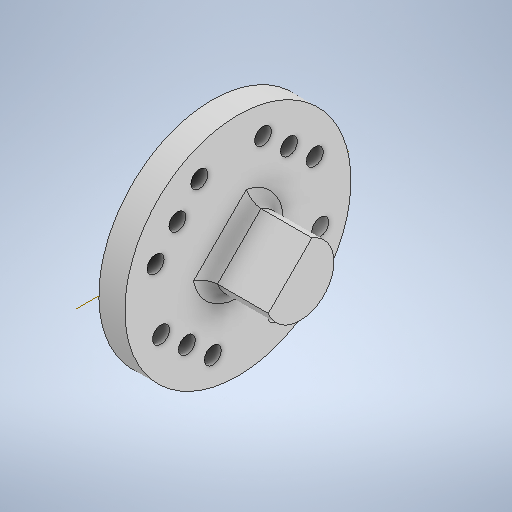
# Autodesk Inventor part: Printed Horn
Saved by Autodesk Inventor 2025.2 (Build 292293000, 293)
## iProperties
Created: 2025-04-05
Part Number: Printed Horn
Material: Generic
Document SubType Name: Modeling
Designer: abdal
Density: 1 g/cm^3
Appearance: Default
Author: abdal
Autodesk Inventor part; units mm, degrees
ref_plane "YZ Plane" through (0, 0, 0) normal (1, 0, 0) x (0, 1, 0)
ref_plane "XZ Plane" through (0, 0, 0) normal (0, 1, 0) x (-1, 0, 0)
ref_plane "XY Plane" through (0, 0, 0) normal (0, 0, 1) x (1, 0, 0)
sketch "Sketch1" plane through (0, 0, 0) normal (1, 0, 0) x (0, 1, 0)
  circle A0 centre (0, 0) radius 10
  dimension "d0" = 20
  constraints: 1 centre point, 1 coincident
  measures "d0" diameter of A0
extrude "Extrusion1" add sketch "Sketch1" along normal blind 2.3
sketch "Sketch2" plane through (2.3, 0, 0) normal (1, 0, 0) x (0, 0, -1)
  circle A0 centre (0, 0) radius 10 projected
  circle A1 centre (-5.3514, 4.5124) radius 0.75 projected
  circle A2 centre (-7.2853, 2.219) radius 0.75 projected
  circle A3 centre (-4.5124, -5.3514) radius 0.75 projected
  circle A4 centre (-2.219, -7.2853) radius 0.75 projected
  circle A5 centre (3.4175, -6.8059) radius 0.75 projected
  circle A6 centre (4.5124, 5.3514) radius 0.75 projected
  circle A7 centre (2.219, 7.2853) radius 0.75 projected
  circle A8 centre (0, 0) radius 4.4 projected
  circle A9 centre (6.8059, 3.4175) radius 0.75 projected
  circle A10 centre (7.2853, -2.219) radius 0.75 projected
  circle A11 centre (5.3514, -4.5124) radius 0.75 projected
  circle A12 centre (-6.8059, -3.4175) radius 0.75 projected
  circle A13 centre (-3.4175, 6.8059) radius 0.75 projected
  circle A14 centre (0, 0) radius 1.5 projected
  point P0 (0, 0)
extrude "Extrusion2" cut sketch "Sketch2" against normal through all contours A1 | A2 | A3 | A4 | A5 | A6 | A7 | A9 | A10 | A11 | A12 | A13
sketch "Sketch3" plane through (2.3, 0, 0) normal (1, 0, 0) x (0, 0, -1)
  circle A0 centre (0, 0) radius 3
  line L0 (-4.1558, -4.1558) -> (4.1558, 4.1558) construction
  line L1 (14, 0) -> (-14, 0) projected
  line L2 (-2.8123, -1.0445) -> (1.0445, 2.8123)
  point P0 (-0.8839, 0.8839)
  dimension "d5" = 6
  dimension "d6" = 45
  dimension "d7" = 1.25
  constraints: 4 end point, 2 midpoint, 2 point on circle, 1 centre point, 1 coincident, 1 parallel
  measures "d5" diameter of A0
  measures "d6" angle of L1 L0
  measures "d7" distance of point (-0.884, 0.884) point (0, 0)
extrude "Extrusion3" add sketch "Sketch3" along normal blind 5.5 contours L1 L2 A0 | A0 L2 L1 picked at (1.3813, 0.2407) picked at (1.3839, -0.2301)
fillet "Fillet1" radius 1 2 edges at (2.3, 0.8839, 0.8839) (2.3, -2.1213, -2.1213)
body "Solid1"
